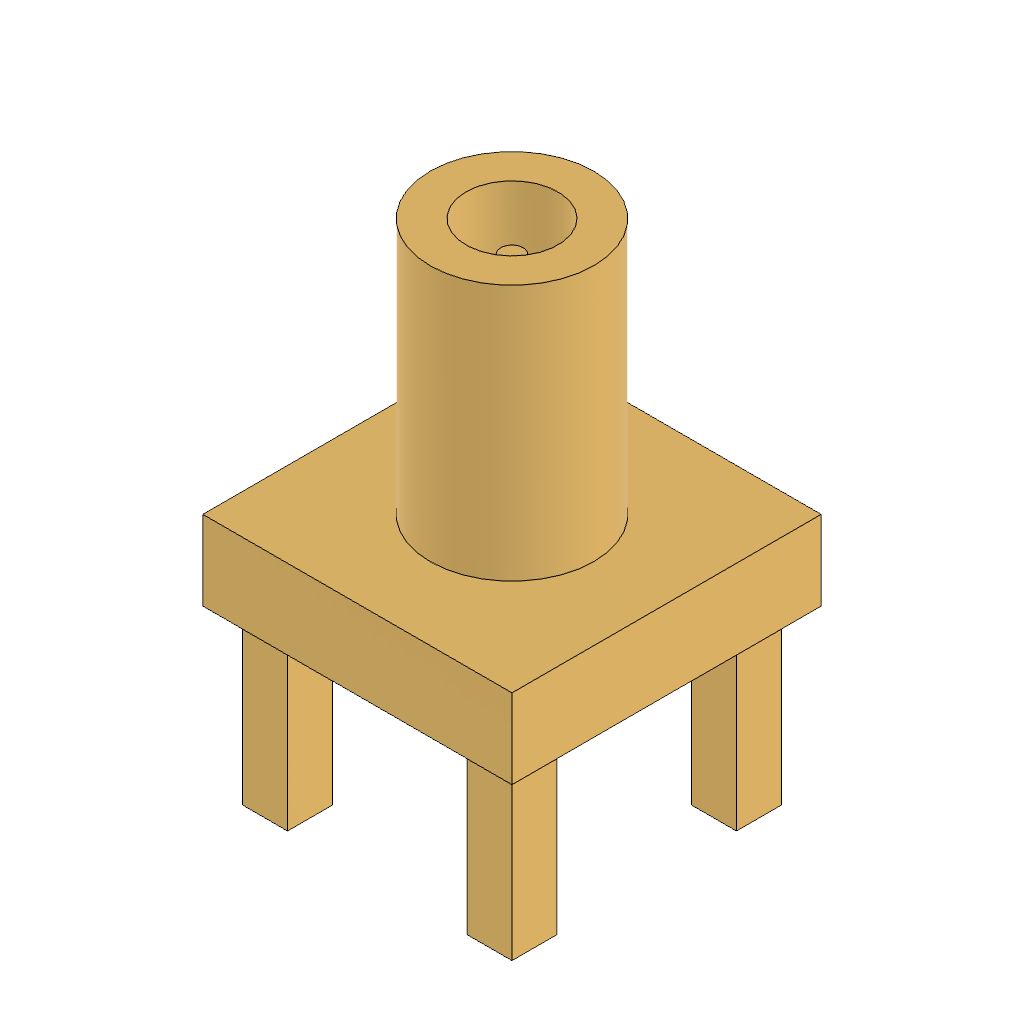
Amphenol_RF_142138_Drawing_Reconstruction (Autodesk Fusion 360 design; units mm, degrees)
description: Manufacturer Rev B mounting dimensions; no scaled SMA. Undimensioned mating barrel/internal details are visual references. See provenance JSON.
part number: 142138
description: 7 x 7 x 7.6 mm conservative nominal upper envelope within the drawing base footprint; excludes tolerances, mated cable and solder tails.
part number: REF-142138-UPPER-ENVELOPE
Autodesk Fusion 360 part; units mm, degrees
ref_plane "WorkPlane1" through (0, 0, 0) normal (0, 0, 1) x (1, 0, 0) in component "Amphenol RF 142138 - drawing reconstruction; mating details reference"
sketch "7 mm square base profile" plane through (0, 0, 0) normal (0, 0, 1) x (1, 0, 0) in component "Amphenol RF 142138 - drawing reconstruction; mating details reference"
  line L0 (-3.5, -3.5) -> (3.5, -3.5)
  line L1 (3.5, -3.5) -> (3.5, 3.5)
  line L2 (3.5, 3.5) -> (-3.5, 3.5)
  line L3 (-3.5, 3.5) -> (-3.5, -3.5)
  dimension "d17" = 3.5
  dimension "d18" = 3.5
  dimension "d19" = 7
  dimension "d20" = 7
  constraint horizontal L0
  constraint vertical L1
  constraint horizontal L2
  constraint vertical L3
  measures "d17" horizontal distance of origin L0.start
  measures "d18" vertical distance of origin L0.start
  measures "d19" horizontal distance of L0.start L0.end
  measures "d20" vertical distance of L0.end L1.end
extrude "7 mm square base" add sketch "7 mm square base profile" along normal blind 1.8 makes body 1 in component "Amphenol RF 142138 - drawing reconstruction; mating details reference"
ref_plane "WorkPlane2" through (0, 0, -3.9) normal (0, 0, 1) x (1, 0, 0) in component "Amphenol RF 142138 - drawing reconstruction; mating details reference"
sketch "Drawing square shell leg -1 -1 profile" plane through (0, 0, -3.9) normal (0, 0, 1) x (1, 0, 0) in component "Amphenol RF 142138 - drawing reconstruction; mating details reference"
  line L0 (-3.05, -3.05) -> (-2.03, -3.05)
  line L1 (-2.03, -3.05) -> (-2.03, -2.03)
  line L2 (-2.03, -2.03) -> (-3.05, -2.03)
  line L3 (-3.05, -2.03) -> (-3.05, -3.05)
  dimension "d25" = 3.05
  dimension "d26" = 3.05
  dimension "d27" = 1.02
  dimension "d28" = 1.02
  constraint horizontal L0
  constraint vertical L1
  constraint horizontal L2
  constraint vertical L3
  measures "d25" horizontal distance of origin L0.start
  measures "d26" vertical distance of origin L0.start
  measures "d27" horizontal distance of L0.start L0.end
  measures "d28" vertical distance of L0.end L1.end
extrude "Drawing square shell leg -1 -1" add sketch "Drawing square shell leg -1 -1 profile" along normal blind 3.9 bodies 1 in component "Amphenol RF 142138 - drawing reconstruction; mating details reference"
ref_plane "WorkPlane3" through (0, 0, -3.9) normal (0, 0, 1) x (1, 0, 0) in component "Amphenol RF 142138 - drawing reconstruction; mating details reference"
sketch "Drawing square shell leg -1 1 profile" plane through (0, 0, -3.9) normal (0, 0, 1) x (1, 0, 0) in component "Amphenol RF 142138 - drawing reconstruction; mating details reference"
  line L0 (-3.05, 2.03) -> (-2.03, 2.03)
  line L1 (-2.03, 2.03) -> (-2.03, 3.05)
  line L2 (-2.03, 3.05) -> (-3.05, 3.05)
  line L3 (-3.05, 3.05) -> (-3.05, 2.03)
  dimension "d33" = 3.05
  dimension "d34" = 2.03
  dimension "d35" = 1.02
  dimension "d36" = 1.02
  constraint horizontal L0
  constraint vertical L1
  constraint horizontal L2
  constraint vertical L3
  measures "d33" horizontal distance of origin L0.start
  measures "d34" vertical distance of origin L0.start
  measures "d35" horizontal distance of L0.start L0.end
  measures "d36" vertical distance of L0.end L1.end
extrude "Drawing square shell leg -1 1" add sketch "Drawing square shell leg -1 1 profile" along normal blind 3.9 bodies 1 in component "Amphenol RF 142138 - drawing reconstruction; mating details reference"
ref_plane "WorkPlane4" through (0, 0, -3.9) normal (0, 0, 1) x (1, 0, 0) in component "Amphenol RF 142138 - drawing reconstruction; mating details reference"
sketch "Drawing square shell leg 1 -1 profile" plane through (0, 0, -3.9) normal (0, 0, 1) x (1, 0, 0) in component "Amphenol RF 142138 - drawing reconstruction; mating details reference"
  line L0 (2.03, -3.05) -> (3.05, -3.05)
  line L1 (3.05, -3.05) -> (3.05, -2.03)
  line L2 (3.05, -2.03) -> (2.03, -2.03)
  line L3 (2.03, -2.03) -> (2.03, -3.05)
  dimension "d41" = 2.03
  dimension "d42" = 3.05
  dimension "d43" = 1.02
  dimension "d44" = 1.02
  constraint horizontal L0
  constraint vertical L1
  constraint horizontal L2
  constraint vertical L3
  measures "d41" horizontal distance of origin L0.start
  measures "d42" vertical distance of origin L0.start
  measures "d43" horizontal distance of L0.start L0.end
  measures "d44" vertical distance of L0.end L1.end
extrude "Drawing square shell leg 1 -1" add sketch "Drawing square shell leg 1 -1 profile" along normal blind 3.9 bodies 1 in component "Amphenol RF 142138 - drawing reconstruction; mating details reference"
ref_plane "WorkPlane5" through (0, 0, -3.9) normal (0, 0, 1) x (1, 0, 0) in component "Amphenol RF 142138 - drawing reconstruction; mating details reference"
sketch "Drawing square shell leg 1 1 profile" plane through (0, 0, -3.9) normal (0, 0, 1) x (1, 0, 0) in component "Amphenol RF 142138 - drawing reconstruction; mating details reference"
  line L0 (2.03, 2.03) -> (3.05, 2.03)
  line L1 (3.05, 2.03) -> (3.05, 3.05)
  line L2 (3.05, 3.05) -> (2.03, 3.05)
  line L3 (2.03, 3.05) -> (2.03, 2.03)
  dimension "d49" = 2.03
  dimension "d50" = 2.03
  dimension "d51" = 1.02
  dimension "d52" = 1.02
  constraint horizontal L0
  constraint vertical L1
  constraint horizontal L2
  constraint vertical L3
  measures "d49" horizontal distance of origin L0.start
  measures "d50" vertical distance of origin L0.start
  measures "d51" horizontal distance of L0.start L0.end
  measures "d52" vertical distance of L0.end L1.end
extrude "Drawing square shell leg 1 1" add sketch "Drawing square shell leg 1 1 profile" along normal blind 3.9 bodies 1 in component "Amphenol RF 142138 - drawing reconstruction; mating details reference"
ref_plane "WorkPlane6" through (0, 0, 1.8) normal (0, 0, 1) x (1, 0, 0) in component "Amphenol RF 142138 - drawing reconstruction; mating details reference"
sketch "Simplified reference barrel - full profile unverified profile" plane through (0, 0, 1.8) normal (0, 0, 1) x (1, 0, 0) in component "Amphenol RF 142138 - drawing reconstruction; mating details reference"
  circle A0 centre (0, 0) radius 1.8542
  dimension "d57" = 1.8542
  measures "d57" radius of A0
extrude "Simplified reference barrel - full profile unverified" add sketch "Simplified reference barrel - full profile unverified profile" along normal blind 5.8 bodies 1 in component "Amphenol RF 142138 - drawing reconstruction; mating details reference"
ref_plane "WorkPlane7" through (0, 0, 0) normal (0, 0, 1) x (1, 0, 0) in component "Amphenol RF 142138 - drawing reconstruction; mating details reference"
sketch "Reference insulator bore - undimensioned depth profile" plane through (0, 0, 0) normal (0, 0, 1) x (1, 0, 0) in component "Amphenol RF 142138 - drawing reconstruction; mating details reference"
  circle A0 centre (0, 0) radius 1.0414
  dimension "d62" = 1.0414
  measures "d62" radius of A0
extrude "Reference insulator bore - undimensioned depth" cut sketch "Reference insulator bore - undimensioned depth profile" along normal blind 7.6 bodies 1 in component "Amphenol RF 142138 - drawing reconstruction; mating details reference"
ref_plane "WorkPlane8" through (0, 0, -3.9) normal (0, 0, 1) x (1, 0, 0) in component "Amphenol RF 142138 - drawing reconstruction; mating details reference"
sketch "Drawing diameter 0.96 signal solder tail profile" plane through (0, 0, -3.9) normal (0, 0, 1) x (1, 0, 0) in component "Amphenol RF 142138 - drawing reconstruction; mating details reference"
  circle A0 centre (0, 0) radius 0.48
  dimension "d67" = 0.48
  measures "d67" radius of A0
extrude "Drawing diameter 0.96 signal solder tail" add sketch "Drawing diameter 0.96 signal solder tail profile" along normal blind 5.7 separate body makes body 2 in component "Amphenol RF 142138 - drawing reconstruction; mating details reference"
ref_plane "WorkPlane9" through (0, 0, 1.8) normal (0, 0, 1) x (1, 0, 0) in component "Amphenol RF 142138 - drawing reconstruction; mating details reference"
sketch "Reference mating pin - projection unverified profile" plane through (0, 0, 1.8) normal (0, 0, 1) x (1, 0, 0) in component "Amphenol RF 142138 - drawing reconstruction; mating details reference"
  circle A0 centre (0, 0) radius 0.254
  dimension "d72" = 0.254
  measures "d72" radius of A0
extrude "Reference mating pin - projection unverified" add sketch "Reference mating pin - projection unverified profile" along normal blind 5.1 bodies 2 in component "Amphenol RF 142138 - drawing reconstruction; mating details reference"
ref_plane "WorkPlane10" through (0, 0, 0) normal (0, 0, 1) x (1, 0, 0) in component "Amphenol RF 142138 - drawing reconstruction; mating details reference"
sketch "Reference natural PTFE insulator profile" plane through (0, 0, 0) normal (0, 0, 1) x (1, 0, 0) in component "Amphenol RF 142138 - drawing reconstruction; mating details reference"
  circle A0 centre (0, 0) radius 1.0364
  dimension "d77" = 1.0364
  measures "d77" radius of A0
extrude "Reference natural PTFE insulator" add sketch "Reference natural PTFE insulator profile" along normal blind 5.8 separate body makes body 3 in component "Amphenol RF 142138 - drawing reconstruction; mating details reference"
ref_plane "WorkPlane11" through (0, 0, 0) normal (0, 0, 1) x (1, 0, 0) in component "Amphenol RF 142138 - drawing reconstruction; mating details reference"
sketch "Reference insulator centre relief profile" plane through (0, 0, 0) normal (0, 0, 1) x (1, 0, 0) in component "Amphenol RF 142138 - drawing reconstruction; mating details reference"
  circle A0 centre (0, 0) radius 0.485
  dimension "d82" = 0.485
  measures "d82" radius of A0
extrude "Reference insulator centre relief" cut sketch "Reference insulator centre relief profile" along normal blind 5.8 bodies 3 in component "Amphenol RF 142138 - drawing reconstruction; mating details reference"
ref_plane "WorkPlane1" through (0, 0, 0) normal (0, 0, 1) x (1, 0, 0) in component "142138 nominal upper occupied-space envelope - no mating geometry"
sketch "Nominal 7 x 7 x 7.6 upper envelope profile" plane through (0, 0, 0) normal (0, 0, 1) x (1, 0, 0) in component "142138 nominal upper occupied-space envelope - no mating geometry"
  line L0 (-3.5, -3.5) -> (3.5, -3.5)
  line L1 (3.5, -3.5) -> (3.5, 3.5)
  line L2 (3.5, 3.5) -> (-3.5, 3.5)
  line L3 (-3.5, 3.5) -> (-3.5, -3.5)
  dimension "d87" = 3.5
  dimension "d88" = 3.5
  dimension "d89" = 7
  dimension "d90" = 7
  constraint horizontal L0
  constraint vertical L1
  constraint horizontal L2
  constraint vertical L3
  measures "d87" horizontal distance of origin L0.start
  measures "d88" vertical distance of origin L0.start
  measures "d89" horizontal distance of L0.start L0.end
  measures "d90" vertical distance of L0.end L1.end
extrude "Nominal 7 x 7 x 7.6 upper envelope" add sketch "Nominal 7 x 7 x 7.6 upper envelope profile" along normal blind 7.6 separate body makes body 4 in component "142138 nominal upper occupied-space envelope - no mating geometry"
component "Amphenol RF 142138 - drawing reconstruction; mating details reference" placed x (1, 0, 0) y (0, 1, 0) z (0, 0, 1) at (0, 0, 0)
component "142138 nominal upper occupied-space envelope - no mating geometry" placed x (1, 0, 0) y (0, 1, 0) z (0, 0, 1) at (0, 0, 0)
equation "BaseSide = 7 mm" comment "Rev B: square base side."
equation "OverallLength = 11.5 mm" comment "Rev B: nose to tail tip."
equation "TailProjection = 3.9 mm" comment "Rev B: PCB seating plane to tail tip."
equation "BarrelLength = 5.8 mm" comment "Rev B: front base face to nose."
equation "BaseThickness = OverallLength - TailProjection - BarrelLength" comment "Derived, not independently toleranced: 1.8 mm."
equation "AbovePCB = OverallLength - TailProjection" comment "Derived nominal above-PCB height: 7.6 mm."
equation "ShellPitch = 5.08 mm" comment "Rev B: square shell-leg centre pitch."
equation "ShellLegSide = 1.02 mm" comment "Rev B: four square shell legs."
equation "SignalTailDiameter = 0.96 mm" comment "Rev B: signal solder tail diameter."
equation "BarrelReferenceDiameter = 3.7084 mm" comment "REFERENCE ONLY. Generic SMB interface maximum, extended as a simplified visual barrel; complete 142138 profile is undimensioned."
equation "BoreReferenceDiameter = 2.0828 mm" comment "REFERENCE ONLY. Generic SMB interface minimum; axial bore extent is unverified."
equation "MatingPinReferenceDiameter = 0.508 mm" comment "REFERENCE ONLY. Midpoint of generic SMB .019-.021 inch pin range."
equation "MatingPinReferenceTop = 6.9 mm" comment "REFERENCE ONLY. Pin projection not dimensioned by Rev B; not a mating/clearance datum."
equation "InsulatorReferenceTop = 5.8 mm" comment "REFERENCE ONLY. Internal PTFE extent not dimensioned by Rev B."
equation "d17 = -( -BaseSide / 2 )"
equation "d18 = -( -BaseSide / 2 )"
equation "d19 = BaseSide"
equation "d20 = BaseSide"
equation "d21 = BaseThickness"
equation "d23 = -TailProjection"
equation "d25 = -( -1 * ShellPitch / 2 - ShellLegSide / 2 )"
equation "d26 = -( -1 * ShellPitch / 2 - ShellLegSide / 2 )"
equation "d27 = ShellLegSide"
equation "d28 = ShellLegSide"
equation "d29 = TailProjection"
equation "d31 = -TailProjection"
equation "d33 = -( -1 * ShellPitch / 2 - ShellLegSide / 2 )"
equation "d34 = 1 * ShellPitch / 2 - ShellLegSide / 2"
equation "d35 = ShellLegSide"
equation "d36 = ShellLegSide"
equation "d37 = TailProjection"
equation "d39 = -TailProjection"
equation "d41 = 1 * ShellPitch / 2 - ShellLegSide / 2"
equation "d42 = -( -1 * ShellPitch / 2 - ShellLegSide / 2 )"
equation "d43 = ShellLegSide"
equation "d44 = ShellLegSide"
equation "d45 = TailProjection"
equation "d47 = -TailProjection"
equation "d49 = 1 * ShellPitch / 2 - ShellLegSide / 2"
equation "d50 = 1 * ShellPitch / 2 - ShellLegSide / 2"
equation "d51 = ShellLegSide"
equation "d52 = ShellLegSide"
equation "d53 = TailProjection"
equation "d55 = BaseThickness"
equation "d57 = BarrelReferenceDiameter / 2"
equation "d58 = BarrelLength"
equation "d62 = BoreReferenceDiameter / 2"
equation "d63 = AbovePCB"
equation "d65 = -TailProjection"
equation "d67 = SignalTailDiameter / 2"
equation "d68 = TailProjection + BaseThickness"
equation "d70 = BaseThickness"
equation "d72 = MatingPinReferenceDiameter / 2"
equation "d73 = MatingPinReferenceTop - BaseThickness"
equation "d77 = ( BoreReferenceDiameter - 0.01 mm ) / 2"
equation "d78 = InsulatorReferenceTop"
equation "d82 = ( SignalTailDiameter + 0.01 mm ) / 2"
equation "d83 = InsulatorReferenceTop"
equation "d87 = -( -BaseSide / 2 )"
equation "d88 = -( -BaseSide / 2 )"
equation "d89 = BaseSide"
equation "d90 = BaseSide"
equation "d91 = AbovePCB"
named bodies: "Brass shell and four 1.02 mm square tails - barrel profile reference", "Signal contact - exact solder tail; mating end reference", "PTFE insulator reference - internal dimensions unverified", "Reference upper envelope - nominal dimensions only"
